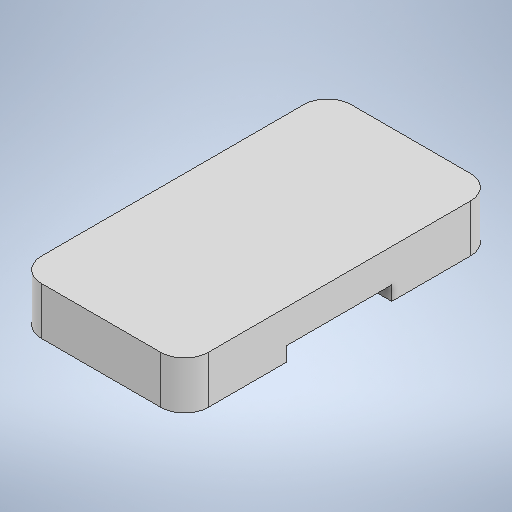
# Autodesk Inventor part: ESC BASE
Saved by Autodesk Inventor 2025 (Build 290162000, 162)
## iProperties
Created: 2024-09-28
Part Number: ESC BASE
Material: Genérico
Document SubType Name: Modeling
Designer: phmca
Density: 1 g/cm^3
Appearance: Padrão
Author: phmca
Autodesk Inventor part; units mm, degrees
ref_plane "YZ Plane" through (0, 0, 0) normal (1, 0, 0) x (0, 1, 0)
ref_plane "XZ Plane" through (0, 0, 0) normal (0, 1, 0) x (-1, 0, 0)
ref_plane "XY Plane" through (0, 0, 0) normal (0, 0, 1) x (1, 0, 0)
sketch "Esboço1" plane through (0, 0, 0) normal (0, 1, 0) x (-1, 0, 0)
  line L0 (17.5, 32.5) -> (-17.5, 32.5)
  line L1 (-17.5, 32.5) -> (-17.5, -32.5)
  line L2 (-17.5, -32.5) -> (17.5, -32.5)
  line L3 (17.5, -32.5) -> (17.5, 32.5)
  line L4 (17.5, 32.5) -> (-17.5, -32.5) construction
  line L5 (-17.5, 32.5) -> (17.5, -32.5) construction
  point P0 (0, 0)
  dimension "d0" = 35
  dimension "d1" = 65
  constraints: 12 end point, 2 midpoint, 2 parallel, 1 horizontal, 1 perpendicular
  measures "d0" distance of L1.end L2.end
  measures "d1" distance of L0.end L1.end
extrude "Extrusão1" add sketch "Esboço1" along normal blind 10
fillet "Arredondamento1" radius 5 4 edges at (17.5, 5, 32.5) (-17.5, 5, 32.5) (17.5, 5, -32.5) (-17.5, 5, -32.5)
sketch "Esboço2" plane through (-17.5, 0, -27.5) normal (-1, 0, 0) x (0, 0, 1)
  line L0 (16.5, -3) -> (38.5, -3)
  line L1 (38.5, -3) -> (38.5, 3)
  line L2 (38.5, 3) -> (16.5, 3)
  line L3 (16.5, 3) -> (16.5, -3)
  line L4 (16.5, -3) -> (38.5, 3) construction
  line L5 (38.5, -3) -> (16.5, 3) construction
  point P0 (27.5, 0)
  dimension "d5" = 22
  dimension "d6" = 6
  constraints: 12 end point, 2 midpoint, 2 parallel, 1 horizontal, 1 perpendicular
  measures "d5" distance of L1.end L2.end
  measures "d6" distance of L0.end L1.end
extrude "Extrusão2" cut sketch "Esboço2" against normal up to surface (35 mm away)
